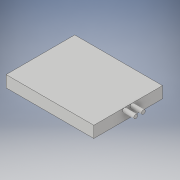
# Autodesk Inventor part: Battery
Saved by Autodesk Inventor 2017 (Build 210142000, 142)
## iProperties
Created: 2017-03-19
Part Number: Battery
Material: Generic
Document SubType Name: Modeling
Designer: Liam
Density: 1 g/cm^3
Appearance: Default
Author: Liam
Autodesk Inventor part; units mm, degrees
ref_plane "YZ Plane" through (0, 0, 0) normal (1, 0, 0) x (0, 1, 0)
ref_plane "XZ Plane" through (0, 0, 0) normal (0, 1, 0) x (-1, 0, 0)
ref_plane "XY Plane" through (0, 0, 0) normal (0, 0, 1) x (1, 0, 0)
sketch "Sketch1" plane through (0, 0, 0) normal (0, 1, 0) x (-1, 0, 0)
  line L0 (0, 0) -> (36.5125, 0)
  line L1 (36.5125, 0) -> (36.5125, -28.575)
  line L2 (36.5125, -28.575) -> (0, -28.575)
  line L3 (0, -28.575) -> (0, 0)
  dimension "d0" = 36.5125
  dimension "d1" = 28.575
  constraints: 8 end point, 2 parallel, 1 horizontal, 1 perpendicular
  measures "d0" distance of L1.end L2.end
  measures "d1" distance of L0.end L1.end
extrude "Extrusion1" add sketch "Sketch1" along normal blind 4.7625
sketch "Sketch3" plane through (0, 0, 0) normal (1, 0, 0) x (0, 0, -1)
  circle A0 centre (12.7, 3.9688) radius 0.7937
  line L0 (0, 4.7625) -> (28.575, 4.7625) projected
  line L1 (0, 0) -> (0, 4.7625) projected
  circle A1 centre (15.875, 3.9688) radius 0.7937
  line L2 (28.575, 0) -> (28.575, 4.7625) projected
  dimension "d5" = 12.7
  dimension "d7" = 12.7
  dimension "d10" = 1.5875
  dimension "d11" = 1.5875
  constraints: 2 centre point, 2 tangent
  measures "d5" distance from line of L1 A0.centre
  measures "d7" distance from line of L2 A1.centre
  measures "d10" diameter of A0
  measures "d11" diameter of A1
extrude "Extrusion2" add sketch "Sketch3" along normal blind 4.7625
body "Solid1"
